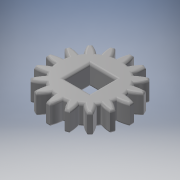
# Autodesk Inventor part: Spur Gear1
Saved by Autodesk Inventor 2017 (Build 210142000, 142)
## iProperties
CustomPartVersion: 1
Created: 2017-08-19
Part Number: Spur Gear1
Material: Steel
Document SubType Name: Modeling
Designer: Dale
Categories: <?xml version="1.0" encoding="UTF-16"?> <MemberInstance><Categories><FamilyTemplate><FamilyTemplateParameter ValueType="xs:double" Id="1" ObjectReferenceKey="da_z" ObjectType="kUserParameterObject"/><FamilyTemplateParameter ValueType="xs:double" Id="2" ObjectReferenceKey="da_b" ObjectType="kUserParameterObject"/><FamilyTemplateParameter ValueType="xs:double" Id="3" ObjectReferenceKey="da_beta" ObjectType="kUserParameterObject"/><FamilyTemplateParameter ValueType="xs:double" Id="4" ObjectReferenceKey="da_da" ObjectType="kUserParameterObject"/><FamilyTemplateParameter ValueType="xs:double" Id="5" ObjectReferenceKey="da_aw" ObjectType="kUserParameterObject"/><FamilyTemplateParameter ValueType="xs:string" Id="6" ObjectReferenceKey="EAIAABAAAACIAQAAAAAAAIAAAAAAAAAA" ObjectType="83910656" SubObjectId="SurfaceGeometry"/></FamilyTemplate><ParamToTemplateMap><ParamToTemplate CategoryParameter="//CategoryParameter[@InternalName='046C89C9-8512-4d59-83FE-43B91F4F132A']" TemplateParameter="1"/><ParamToTemplate CategoryParameter="//CategoryParameter[@InternalName='2552DF32-E462-4b46-AEBF-C6C7768E72AC']" TemplateParameter="2"/><ParamToTemplate CategoryParameter="//CategoryParameter[@InternalName='C9EE641D-15FC-4fae-A226-E94C4372FDD7']" TemplateParameter="3"/><ParamToTemplate><ParamToTemplate CategoryParameter="//CategoryParameter[@InternalName='00B6519A-459B-49c7-AD84-2E56D39A5744']" ConstantValue="0.000000"/></ParamToTemplate><ParamToTemplate><ParamToTemplate CategoryParameter="//CategoryParameter[@InternalName='04B31F0E-C7A6-4894-AA32-9629BEFACF47']" ConstantValue="1.000000"/></ParamToTemplate><ParamToTemplate><ParamToTemplate CategoryParameter="//CategoryParameter[@InternalName='43CBEC2E-7847-49e7-A936-2F7889FCB2D9']" ConstantValue="0.250000"/></ParamToTemplate><ParamToTemplate><ParamToTemplate CategoryParameter="//CategoryParameter[@InternalName='B1EFC894-105D-4ebd-86BF-FA20ED196853']" ConstantValue="0.350000"/></ParamToTemplate><ParamToTemplate><ParamToTemplate CategoryParameter="//CategoryParameter[@InternalName='51175063-3D10-4879-93E8-6246FE8B403D']" ConstantValue="2060000000.000000"/></ParamToTemplate><ParamToTemplate><ParamToTemplate CategoryParameter="//CategoryParameter[@InternalName='A3A52E27-4454-46a9-B0BD-C932399B70AF']" ConstantValue="0.300000"/></ParamToTemplate><ParamToTemplate><ParamToTemplate CategoryParameter="//CategoryParameter[@InternalName='91B76062-C214-41d9-B1B9-14D2AB99603D']" ConstantValue="0.181429"/></ParamToTemplate><ParamToTemplate><ParamToTemplate CategoryParameter="//CategoryParameter[@InternalName='374E806E-8B8A-4dda-A9AA-1039D6500AD2']" ConstantValue="5.511811"/></ParamToTemplate><ParamToTemplate><ParamToTemplate CategoryParameter="//CategoryParameter[@InternalName='2D373A89-B862-43d6-8D0B-0CBF12AB9F6C']" ConstantValue="0.349066"/></ParamToTemplate><ParamToTemplate CategoryParameter="//CategoryParameter[@InternalName='37777632-D6A2-4fac-9D53-DB8ACD95C989']" TemplateParameter="4"/><ParamToTemplate CategoryParameter="//CategoryParameter[@InternalName='FD1017F1-B727-4f7e-9707-0F86F1FF9423']" TemplateParameter="5"/><ParamToTemplate><ParamToTemplate CategoryParameter="//CategoryParameter[@InternalName='9E1B4470-B2D3-4ff1-B813-535BB4CDF51A']" ConstantValue="3520000.000000"/></ParamToTemplate><ParamToTemplate><ParamToTemplate CategoryParameter="//CategoryParameter[@InternalName='F8452263-BFF6-458c-9FB1-07C4B99E95CD']" ConstantValue="11400000.000000"/></ParamToTemplate><ParamToTemplate><ParamToTemplate CategoryParameter="//CategoryParameter[@InternalName='3E3BB259-FD49-497f-8171-6EBC954A3479']" ConstantValue="2.000000"/></ParamToTemplate><ParamToTemplate CategoryParameter="//CategoryParameter[@InternalName='27C3BAF2-7550-4e4b-AE2C-0DB134B7D9B7']" TemplateParameter="6"/></ParamToTemplateMap><Category DisplayName="Gear" InternalName="DC85795E-93AB-48d5-8EEE-5A27447B64BD" Mnemonic="Gear"><CategoryParameter DisplayName="z" InternalName="046C89C9-8512-4d59-83FE-43B91F4F132A" Mnemonic="z"/><CategoryParameter DisplayName="b" InternalName="2552DF32-E462-4b46-AEBF-C6C7768E72AC" Mnemonic="b"/><CategoryParameter DisplayName="||b|" InternalName="C9EE641D-15FC-4fae-A226-E94C4372FDD7" Mnemonic="beta"/><CategoryParameter DisplayName="x" InternalName="00B6519A-459B-49c7-AD84-2E56D39A5744" Mnemonic="x"/><CategoryParameter DisplayName="a*" InternalName="04B31F0E-C7A6-4894-AA32-9629BEFACF47" Mnemonic="a"/><CategoryParameter DisplayName="c*" InternalName="43CBEC2E-7847-49e7-A936-2F7889FCB2D9" Mnemonic="c"/><CategoryParameter DisplayName="r|.f|*" InternalName="B1EFC894-105D-4ebd-86BF-FA20ED196853" Mnemonic="rf"/><CategoryParameter DisplayName="E" InternalName="51175063-3D10-4879-93E8-6246FE8B403D" Mnemonic="E"/><CategoryParameter DisplayName="||m|" InternalName="A3A52E27-4454-46a9-B0BD-C932399B70AF" Mnemonic="mi"/><Category DisplayName="SpurGear" InternalName="26C5A22E-A91E-4dfd-A3B3-23CCAFAE1764" Mnemonic="SpurGear"><CategoryParameter DisplayName="m" InternalName="91B76062-C214-41d9-B1B9-14D2AB99603D" Mnemonic="m"/><CategoryParameter DisplayName="P" InternalName="374E806E-8B8A-4dda-A9AA-1039D6500AD2" Mnemonic="PP"/><CategoryParameter DisplayName="||a|" InternalName="2D373A89-B862-43d6-8D0B-0CBF12AB9F6C" Mnemonic="alpha"/><CategoryParameter DisplayName="d|.a|" InternalName="37777632-D6A2-4fac-9D53-DB8ACD95C989" Mnemonic="da"/><CategoryParameter DisplayName="a|.w|" InternalName="FD1017F1-B727-4f7e-9707-0F86F1FF9423" Mnemonic="aw"/><CategoryParameter DisplayName="||s||.Flim|" InternalName="9E1B4470-B2D3-4ff1-B813-535BB4CDF51A" Mnemonic="sFlim"/><CategoryParameter DisplayName="||s||.Hlim|" InternalName="F8452263-BFF6-458c-9FB1-07C4B99E95CD" Mnemonic="sHlim"/><CategoryParameter DisplayName="type" InternalName="3E3BB259-FD49-497f-8171-6EBC954A3479" Mnemonic="type"/><CategoryParameter DisplayName="PitchDiameter" InternalName="27C3BAF2-7550-4e4b-AE2C-0DB134B7D9B7" Mnemonic="IDS_PITCHDIAM"/></Category></Category></Categories></MemberInstance>
Density: 1 g/cm^3
Appearance: Steel
Author: Dale
## iProperties of the stored document Spur Gear1_3DPrint.ipt
Created: 2017-08-19
Part Number: Spur Gear1_3DPrint
Material: Generic
Document SubType Name: Modeling
Designer: Dale
Density: 1 g/cm^3
Appearance: Default
Author: Dale
Autodesk Inventor part; units mm, degrees
sketch "Sketch1" plane through (0, 0, 0) normal (0, 0, 1) x (1, 0, 0)
  circle A0 centre (0, 0) radius 16.3286
  dimension "d0" = 32.6571
  constraints: 1 centre point
  measures "d0" diameter of A0
extrude "Extrusion1" add sketch "Sketch1" along normal blind 8
ref_plane "Work Plane2" through (0, 0, 4) normal (0, 0, 1) x (1, 0, 0)
sketch "Sketch2" plane through (0, 0, 0) normal (0, 0, -1) x (-1, 0, 0)
  circle A0 centre (0, 0) radius 16.3286 projected
  circle A1 centre (0, 0) radius 14.5143
  dimension "d3" = 29.0286
  constraints: 1 centre point, 1 coincident
  measures "d3" diameter of A1
surface extrude "Pitch Diameter" sketch "Sketch2" against normal through all shown no curves A1
ref_plane "Work Plane8" through (0, 0, 0) normal (0.9807853, 0.1950903, 0) x (0, 0, 1)
ref_plane "Work Plane9" through (0, 0, 0) normal (1, 0, 0) x (0, 1, 0)
spur gear teeth "Spur Gear" teeth 16 pitch diameter 29.0286 tip diameter 32.6571 root diameter 24.4929 face width 8 start plane through (0, 0, 0) normal (0, 0, -1) x (-1, 0, 0)
sketch "Sketch3" plane through (0, 0, 8) normal (0, 0, 1) x (1, 0, 0)
  line L0 (-4.95, 4.95) -> (4.95, 4.95)
  line L1 (4.95, 4.95) -> (4.95, -4.95)
  line L2 (4.95, -4.95) -> (-4.95, -4.95)
  line L3 (-4.95, -4.95) -> (-4.95, 4.95)
  point P0 (0, 0)
  point P1 (4.95, 0)
  point P2 (0, 4.95)
  dimension "d49" = 9.9
  constraints: 8 end point, 2 midpoint, 2 parallel, 2 perpendicular, 1 horizontal, 1 horizontal alignment, 1 vertical alignment
  measures "d49" distance of L0.start L0.end
extrude "Shaft Cutout" cut sketch "Sketch3" against normal up to next
fillet "Shaft Edges" radius 1 8 edges at (-4.95, 0, 8) (0, 4.95, 8) (4.95, 0, 8) (0, -4.95, 8) (-4.95, 0, 0) (0, 4.95, 0) (4.95, 0, 0) (0, -4.95, 0)
fillet "Edge Bevels" radius 1 128 edges at (-11.117, -9.0383, 8) (0, 16.3286, 8) (6.2487, 15.0856, 8) (11.546, 11.546, 8) (15.0856, 6.2487, 8) (16.3286, 0, 8) (15.0856, -6.2487, 8) (11.546, -11.546, 8) (6.2487, -15.0856, 8) (0, -16.3286, 8) (-6.2487, -15.0856, 8) (-11.546, -11.546, 8) (-15.0856, -6.2487, 8) (-16.3286, 0, 8) (-15.0856, 6.2487, 8) (-11.546, 11.546, 8) (-6.2487, 15.0856, 8) (-6.8119, 12.6046, 8) (-6.8038, 10.1825, 8) (-9.0383, 11.117, 8) (-11.117, 9.0383, 8) (-10.1825, 6.8038, 8) (-12.6046, 6.8119, 8) (-13.7296, 4.096, 8) (-12.0111, 2.3892, 8) (-14.2519, 1.4698, 8) (-14.2519, -1.4698, 8) (-12.0111, -2.3892, 8) (-13.7296, -4.096, 8) (-12.6046, -6.8119, 8) (-10.1825, -6.8038, 8) (-9.0383, -11.117, 8) (-6.8038, -10.1825, 8) (-6.8119, -12.6046, 8) (-4.096, -13.7296, 8) (-2.3892, -12.0111, 8) (-1.4698, -14.2519, 8) (1.4698, -14.2519, 8) (2.3892, -12.0111, 8) (4.096, -13.7296, 8) (6.8119, -12.6046, 8) (6.8038, -10.1825, 8) (9.0383, -11.117, 8) (11.117, -9.0383, 8) (10.1825, -6.8038, 8) (12.6046, -6.8119, 8) (13.7296, -4.096, 8) (12.0111, -2.3892, 8) (14.2519, -1.4698, 8) (14.2519, 1.4698, 8) (12.0111, 2.3892, 8) (13.7296, 4.096, 8) (12.6046, 6.8119, 8) (10.1825, 6.8038, 8) (11.117, 9.0383, 8) (9.0383, 11.117, 8) (6.8038, 10.1825, 8) (6.8119, 12.6046, 8) (4.096, 13.7296, 8) (2.3892, 12.0111, 8) (1.4698, 14.2519, 8) (-1.4698, 14.2519, 8) (-2.3892, 12.0111, 8) (-4.096, 13.7296, 8) (0, 16.3286, 0) (6.2487, 15.0856, 0) (11.546, 11.546, 0) (15.0856, 6.2487, 0) (16.3286, 0, 0) (15.0856, -6.2487, 0) (11.546, -11.546, 0) (6.2487, -15.0856, 0) (0, -16.3286, 0) (-6.2487, -15.0856, 0) (-11.546, -11.546, 0) (-15.0856, -6.2487, 0) (-16.3286, 0, 0) (-15.0856, 6.2487, 0) (-11.546, 11.546, 0) (-6.2487, 15.0856, 0) (-4.096, 13.7296, 0) (-2.3892, 12.0111, 0) (-1.4698, 14.2519, 0) (1.4698, 14.2519, 0) (2.3892, 12.0111, 0) (4.096, 13.7296, 0) (6.8119, 12.6046, 0) (6.8038, 10.1825, 0) (9.0383, 11.117, 0) (11.117, 9.0383, 0) (10.1825, 6.8038, 0) (12.6046, 6.8119, 0) (13.7296, 4.096, 0) (12.0111, 2.3892, 0) (14.2519, 1.4698, 0) (14.2519, -1.4698, 0) (12.0111, -2.3892, 0) (13.7296, -4.096, 0) (12.6046, -6.8119, 0) (10.1825, -6.8038, 0) (11.117, -9.0383, 0) (9.0383, -11.117, 0) (6.8038, -10.1825, 0) (6.8119, -12.6046, 0) (4.096, -13.7296, 0) (2.3892, -12.0111, 0) (1.4698, -14.2519, 0) (-1.4698, -14.2519, 0) (-2.3892, -12.0111, 0) (-4.096, -13.7296, 0) (-6.8119, -12.6046, 0) (-6.8038, -10.1825, 0) (-9.0383, -11.117, 0) (-11.117, -9.0383, 0) (-10.1825, -6.8038, 0) (-12.6046, -6.8119, 0) (-13.7296, -4.096, 0) (-12.0111, -2.3892, 0) (-14.2519, -1.4698, 0) (-14.2519, 1.4698, 0) (-12.0111, 2.3892, 0) (-13.7296, 4.096, 0) (-12.6046, 6.8119, 0) (-10.1825, 6.8038, 0) (-11.117, 9.0383, 0) (-9.0383, 11.117, 0) (-6.8038, 10.1825, 0) (-6.8119, 12.6046, 0)
equation "\"d0\" = da_da"
equation "\"d1\" = da_b"
equation "\"d3\" = da_dw"
equation "\"d16\" = da_aw"
equation "\"d43\" = da_aw"
equation "\"d46\" = da_aw"
equation "\"da_da\" = 32.657143"
equation "\"da_b\" = 8"
equation "\"da_dw\" = 29.028571"
equation "\"da_aw\" = 25.4"
body "Solid1"
body "Srf1"
